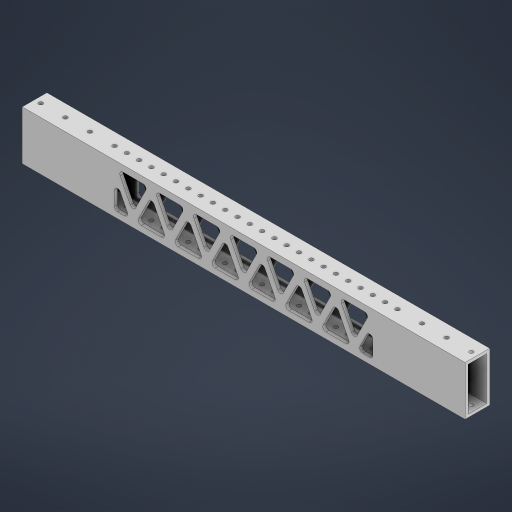
# Autodesk Inventor part: fram_extrusion_18in
Saved by Autodesk Inventor 2023 (Build 270158000, 158)
## iProperties
Created: 2023-02-13
Part Number: fram_extrusion_18in
Material: Generic
Document SubType Name: Modeling
Designer: bryce
Density: 1 g/cm^3
Appearance: Default
Author: bryce
Autodesk Inventor part; units mm, degrees
ref_plane "YZ Plane" through (0, 0, 0) normal (1, 0, 0) x (0, 1, 0)
sketch "Sketch1" plane through (0, 0, 0) normal (1, 0, 0) x (0, 1, 0)
  line L0 (0, 0) -> (50.8, 0)
  line L1 (50.8, 0) -> (50.8, -25.4)
  line L2 (50.8, -25.4) -> (0, -25.4)
  line L3 (0, -25.4) -> (0, 0)
  dimension "d0" = 50.8
  dimension "d1" = 25.4
  constraints: 8 end point, 2 parallel, 1 horizontal, 1 perpendicular
  measures "d0" distance of L1.end L2.end
  measures "d1" distance of L0.end L1.end
extrude "Extrusion1" add sketch "Sketch1" along normal blind 457.2
shell "Shell1" thickness 3.175 removed faces 2 at (0, 16.9333, -16.9333) at (457.2, 16.9333, -16.9333)
sketch "Sketch2" plane through (0, 50.8, 0) normal (0, 1, 0) x (1, 0, 0)
  line L0 (0, 12.7) -> (457.2, 12.7) construction
  line L1 (0, 25.4) -> (0, 0) projected
  circle A0 centre (6.35, 12.7) radius 2.0638
  dimension "d5" = 4.1275
  dimension "d6" = 6.35
  dimension "d7" = 90
  dimension "d8" = 457.2
  constraints: 4 midpoint, 2 end point, 1 centre point, 1 horizontal, 1 point on line
  measures "d5" diameter of A0
  measures "d6" distance of point (0, 12.7) A0.centre
  measures "d7" angle of L1 L0
  measures "d8" distance of L0.start L0.end
hole "Hole1" at (6.35, 50.8, -12.7) direction (0, -1, 0) diameter 4.1275 end through all
pattern_linear "Rectangular Pattern1" count 4 spacing 25.4 along (1, 0, 0) of "Hole1"
ref_plane "Work Plane1" through (228.6, 0, 0) normal (1, 0, 0) x (0, 0, -1)
mirror "Mirror1" about plane through (228.6, 0, 0) normal (1, 0, 0) of "Hole1", "Rectangular Pattern1"
sketch "Sketch3" plane through (0, 50.8, 0) normal (0, 1, 0) x (1, 0, 0)
  circle A0 centre (82.55, 12.7) radius 2.0638 projected
  circle A1 centre (374.65, 12.7) radius 2.0638 projected
  line L0 (82.55, 12.7) -> (374.65, 12.7) construction
  circle A2 centre (95.25, 12.7) radius 2.0637
  point P0 (0, 0)
  dimension "d20" = 4.1275
  dimension "d21" = 12.7
  constraints: 2 end point, 1 centre point, 1 point on line
  measures "d20" diameter of A2
  measures "d21" distance of L0.start A2.centre
hole "Hole2" at (95.25, 50.8, -12.7) direction (0, -1, 0) diameter 4.1275 end through all
pattern_linear "Rectangular Pattern2" count 22 spacing 12.7 along (1, 0, 0) of "Hole2"
sketch "Sketch4" plane through (0, 0, 0) normal (0, 0, 1) x (1, 0, 0)
  line L0 (95.25, 44.45) -> (361.95, 44.45)
  line L1 (361.95, 44.45) -> (361.95, 6.35)
  line L2 (361.95, 6.35) -> (95.25, 6.35)
  line L3 (95.25, 6.35) -> (95.25, 44.45)
  line L4 (0, 50.8) -> (0, 0) projected
  line L5 (457.2, 50.8) -> (457.2, 0) projected
  line L6 (0, 50.8) -> (457.2, 50.8) projected
  line L7 (0, 0) -> (457.2, 0) projected
  dimension "d33" = 95.25
  dimension "d34" = 95.25
  dimension "d35" = 6.35
  dimension "d36" = 6.35
  constraints: 8 end point, 2 parallel, 1 horizontal, 1 perpendicular
  measures "d33" distance between parallel lines of L4 L3
  measures "d34" distance between parallel lines of L5 L1
  measures "d35" distance between parallel lines of L6 L0
  measures "d36" distance between parallel lines of L7 L2
extrude "Extrusion2" cut sketch "Sketch4" against normal up to surface (25.4 mm away) contours L0 L1 L2 L3
sketch "Sketch7" plane through (0, 0, 0) normal (0, 0, 1) x (1, 0, 0)
  line L0 (361.95, 44.45) -> (95.25, 44.45) projected
  line L1 (95.25, 44.45) -> (133.35, 44.45)
  line L2 (114.3, 44.45) -> (114.3, 6.35) construction
  line L3 (95.25, 6.35) -> (361.95, 6.35) projected
  line L4 (95.25, 44.45) -> (114.3, 6.35) construction
  line L5 (133.35, 44.45) -> (114.3, 6.35) construction
  line L6 (92.4102, 43.0301) -> (111.4602, 4.9301)
  line L7 (111.4602, 4.9301) -> (114.3, 6.35)
  line L8 (98.0898, 45.8699) -> (92.4102, 43.0301)
  line L9 (92.4102, 43.0301) -> (117.1398, 7.7699) construction
  line L10 (111.4602, 4.9301) -> (98.0898, 45.8699) construction
  line L11 (130.5102, 45.8699) -> (136.1898, 43.0301)
  line L12 (136.1898, 43.0301) -> (117.1398, 4.9301)
  line L13 (117.1398, 4.9301) -> (114.3, 6.35)
  line L14 (111.4602, 7.7699) -> (136.1898, 43.0301) construction
  line L15 (130.5102, 45.8699) -> (117.1398, 4.9301) construction
  line L16 (117.1398, 7.7699) -> (116.0749, 9.8998)
  line L17 (114.3, 13.4495) -> (98.0898, 45.8699)
  line L18 (114.3, 13.4495) -> (130.5102, 45.8699)
  line L19 (95.25, 44.45) -> (361.95, 44.45) projected
  line L20 (136.8998, 44.45) -> (117.8498, 6.35)
  line L21 (152.4, 13.4495) -> (168.6102, 45.8699)
  line L22 (174.9998, 44.45) -> (155.9498, 6.35)
  line L23 (152.4, 13.4495) -> (136.1898, 45.8699)
  line L24 (130.5102, 43.0301) -> (149.5602, 4.9301)
  line L25 (136.1898, 45.8699) -> (130.5102, 43.0301)
  line L26 (168.6102, 45.8699) -> (174.2898, 43.0301)
  line L27 (149.5602, 4.9301) -> (152.4, 6.35)
  line L28 (155.2398, 4.9301) -> (152.4, 6.35)
  line L29 (174.2898, 43.0301) -> (155.2398, 4.9301)
  line L30 (190.5, 13.4495) -> (206.7102, 45.8699)
  line L31 (213.0998, 44.45) -> (194.0498, 6.35)
  line L32 (190.5, 13.4495) -> (174.2898, 45.8699)
  line L33 (168.6102, 43.0301) -> (187.6602, 4.9301)
  line L34 (174.2898, 45.8699) -> (168.6102, 43.0301)
  line L35 (206.7102, 45.8699) -> (212.3898, 43.0301)
  line L36 (187.6602, 4.9301) -> (190.5, 6.35)
  line L37 (193.3398, 4.9301) -> (190.5, 6.35)
  line L38 (212.3898, 43.0301) -> (193.3398, 4.9301)
  line L39 (228.6, 13.4495) -> (244.8102, 45.8699)
  line L40 (251.1998, 44.45) -> (232.1498, 6.35)
  line L41 (228.6, 13.4495) -> (212.3898, 45.8699)
  line L42 (206.7102, 43.0301) -> (225.7602, 4.9301)
  line L43 (212.3898, 45.8699) -> (206.7102, 43.0301)
  line L44 (244.8102, 45.8699) -> (250.4898, 43.0301)
  line L45 (225.7602, 4.9301) -> (228.6, 6.35)
  line L46 (231.4398, 4.9301) -> (228.6, 6.35)
  line L47 (250.4898, 43.0301) -> (231.4398, 4.9301)
  line L48 (266.7, 13.4495) -> (282.9102, 45.8699)
  line L49 (289.2998, 44.45) -> (270.2498, 6.35)
  line L50 (266.7, 13.4495) -> (250.4898, 45.8699)
  line L51 (244.8102, 43.0301) -> (263.8602, 4.9301)
  line L52 (250.4898, 45.8699) -> (244.8102, 43.0301)
  line L53 (282.9102, 45.8699) -> (288.5898, 43.0301)
  line L54 (263.8602, 4.9301) -> (266.7, 6.35)
  line L55 (269.5398, 4.9301) -> (266.7, 6.35)
  line L56 (288.5898, 43.0301) -> (269.5398, 4.9301)
  line L57 (304.8, 13.4495) -> (321.0102, 45.8699)
  line L58 (327.3998, 44.45) -> (308.3498, 6.35)
  line L59 (304.8, 13.4495) -> (288.5898, 45.8699)
  line L60 (282.9102, 43.0301) -> (301.9602, 4.9301)
  line L61 (288.5898, 45.8699) -> (282.9102, 43.0301)
  line L62 (321.0102, 45.8699) -> (326.6898, 43.0301)
  line L63 (301.9602, 4.9301) -> (304.8, 6.35)
  line L64 (307.6398, 4.9301) -> (304.8, 6.35)
  line L65 (326.6898, 43.0301) -> (307.6398, 4.9301)
  line L66 (342.9, 13.4495) -> (359.1102, 45.8699)
  line L67 (365.4998, 44.45) -> (346.4498, 6.35)
  line L68 (342.9, 13.4495) -> (326.6898, 45.8699)
  line L69 (321.0102, 43.0301) -> (340.0602, 4.9301)
  line L70 (326.6898, 45.8699) -> (321.0102, 43.0301)
  line L71 (359.1102, 45.8699) -> (364.7898, 43.0301)
  line L72 (340.0602, 4.9301) -> (342.9, 6.35)
  line L73 (345.7398, 4.9301) -> (342.9, 6.35)
  line L74 (364.7898, 43.0301) -> (345.7398, 4.9301)
  point P0 (0, 0)
  point P1 (104.775, 25.4)
  point P2 (123.825, 25.4)
  point P3 (129.8002, 44.45)
  point P4 (98.7998, 44.45)
  point P5 (95.25, 44.45)
  point P6 (110.7502, 6.35)
  point P7 (117.8498, 6.35)
  point P8 (133.35, 37.3505)
  point P9 (155.9498, 6.35)
  point P10 (171.45, 37.3505)
  point P11 (194.0498, 6.35)
  point P12 (209.55, 37.3505)
  point P13 (232.1498, 6.35)
  point P14 (247.65, 37.3505)
  point P15 (270.2498, 6.35)
  point P16 (285.75, 37.3505)
  point P17 (308.3498, 6.35)
  point P18 (323.85, 37.3505)
  point P19 (346.4498, 6.35)
  point P20 (323.85, 44.45)
  point P21 (285.75, 44.45)
  point P22 (247.65, 44.45)
  point P23 (209.55, 44.45)
  point P24 (171.45, 44.45)
  dimension "d58" = 38.1
  dimension "d59" = 6.35
  dimension "d60" = 6.35
  dimension "d66" = 38.1
  constraints: 144 end point, 7 midpoint, 6 parallel, 6 point on line, 2 perpendicular, 1 collinear, 1 horizontal, 1 vertical, 114 other
  measures "d58" distance of L0.end L1.end
  measures "d59" distance of L9.end L6.end
  measures "d60" distance of L11.start L11.end
  measures "d66" distance of L17.start L21.start
extrude "Extrusion5" add sketch "Sketch7" against normal up to surface (3.175 mm away) contours L20 L11 L0 | L23 L21 L0 L34 L33 L22 L3 L24 L12 L20 | L0 L25 L23 | L25 L24 L12 L3 L6 L8 L0 L17 L18 | L11 L12 L24 L25 | L21 L26 L0 | L34 L32 L0 | L0 L22 L26 | L26 L22 L33 L34 | L32 L30 L0 L43 L42 L31 L3 L33 L22 | L3 L27 L24 | L30 L35 L0 | L3 L29 L28 | L43 L41 L0 | L0 L31 L35 | L35 L31 L42 L43 | L3 L36 L33 | L41 L39 L0 L52 L51 L40 L3 L42 L31 | L3 L38 L37 | L39 L44 L0 | L52 L50 L0 | L0 L40 L44 | L44 L40 L51 L52 | L3 L45 L42 | L50 L48 L0 L61 L60 L49 L3 L51 L40 | L3 L47 L46 | L48 L53 L0 | L61 L59 L0 | L0 L49 L53 | L53 L49 L60 L61 | L3 L54 L51 | L59 L57 L0 L70 L69 L58 L3 L60 L49 | L3 L56 L55 | L57 L62 L0 | L70 L68 L0 | L0 L58 L62 | L62 L58 L69 L70 | L3 L63 L60 | L68 L66 L0 L71 L67 L3 L69 L58 | L3 L65 L64 | L66 L71 L0 | L3 L72 L69 | L3 L74 L73
fillet "Fillet4" radius 3.175 8 edges at (95.25, 37.3505, -1.5875) (95.25, 6.35, -1.5875) (110.7502, 6.35, -1.5875) (114.3, 13.4495, -1.5875) (98.7998, 44.45, -1.5875) (129.8002, 44.45, -1.5875) (136.8998, 44.45, -1.5875) (117.8498, 6.35, -1.5875)
fillet "Fillet6" radius 3.175 37 edges at (133.35, 37.3505, -1.5875) (148.8502, 6.35, -1.5875) (152.4, 13.4495, -1.5875) (167.9002, 44.45, -1.5875) (171.45, 37.3505, -1.5875) (155.9498, 6.35, -1.5875) (186.9502, 6.35, -1.5875) (190.5, 13.4495, -1.5875) (174.9998, 44.45, -1.5875) (206.0002, 44.45, -1.5875) (209.55, 37.3505, -1.5875) (194.0498, 6.35, -1.5875) (225.0502, 6.35, -1.5875) (213.0998, 44.45, -1.5875) (244.1002, 44.45, -1.5875) (228.6, 13.4495, -1.5875) (232.1498, 6.35, -1.5875) (247.65, 37.3505, -1.5875) (263.1502, 6.35, -1.5875) (266.7, 13.4495, -1.5875) (251.1998, 44.45, -1.5875) (282.2002, 44.45, -1.5875) (270.2498, 6.35, -1.5875) (285.75, 37.3505, -1.5875) (301.2502, 6.35, -1.5875) (289.2998, 44.45, -1.5875) (320.3002, 44.45, -1.5875) (304.8, 13.4495, -1.5875) (308.3498, 6.35, -1.5875) (323.85, 37.3505, -1.5875) (339.3502, 6.35, -1.5875) (342.9, 13.4495, -1.5875) (327.3998, 44.45, -1.5875) (358.4002, 44.45, -1.5875) (361.95, 37.3505, -1.5875) (361.95, 6.35, -1.5875) (346.4498, 6.35, -1.5875)
ref_plane "Work Plane2" through (0, 0, -12.7) normal (0, 0, 1) x (1, 0, 0)
mirror "Mirror2" about plane through (0, 0, -12.7) normal (0, 0, 1) of "Extrusion5", "Fillet4", "Fillet6"
body "Solid1"
